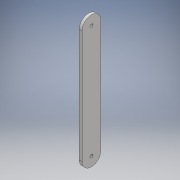
# Autodesk Inventor part: segment1
Saved by Autodesk Inventor 2017 (Build 210142000, 142)
## iProperties
Created: 2017-05-09
Part Number: segment1
Material: Ogólny
Document SubType Name: Modeling
Designer: Damian
Density: 1 g/cm^3
Appearance: Domyślna
Author: Damian
Autodesk Inventor part; units mm, degrees
ref_plane "YZ Plane" through (0, 0, 0) normal (1, 0, 0) x (0, 1, 0)
ref_plane "XZ Plane" through (0, 0, 0) normal (0, 1, 0) x (-1, 0, 0)
ref_plane "XY Plane" through (0, 0, 0) normal (0, 0, 1) x (1, 0, 0)
sketch "Szkic1" plane through (0, 0, 0) normal (1, 0, 0) x (0, 1, 0)
  line L0 (10, 0) -> (10, 0)
  line L1 (20, 10) -> (20, 130)
  line L2 (10, 140) -> (10, 140)
  line L3 (0, 130) -> (0, 10)
  arc A0 (20, 130) -> (10, 140) centre (10, 130) ccw
  arc A1 (10, 140) -> (0, 130) centre (10, 130) ccw
  arc A2 (10, 0) -> (20, 10) centre (10, 10) ccw
  arc A3 (0, 10) -> (10, 0) centre (10, 10) ccw
  circle A4 centre (10, 130) radius 1.6
  circle A5 centre (10, 10) radius 1.6
  point P0 (0, 0)
  point P1 (20, 140)
  point P2 (0, 140)
  dimension "d0" = 20
  dimension "d1" = 10
  dimension "d2" = 10
  dimension "d3" = 10
  dimension "d4" = 10
  dimension "d5" = 3.2
  dimension "d6" = 3.2
  dimension "d7" = 120
  constraints: 8 end point, 8 point on circle, 8 tangent, 6 centre point, 6 point on line, 2 coincident, 2 parallel, 1 horizontal, 1 perpendicular
  measures "d0" distance of point (20, 140) point (0, 140)
  measures "d1" radius of A0
  measures "d2" radius of A1
  measures "d3" radius of A2
  measures "d4" radius of A3
  measures "d5" diameter of A4
  measures "d6" diameter of A5
  measures "d7" distance of A2.centre A0.centre
extrude "Wyciągnięcie proste1" add sketch "Szkic1" along normal blind 3
